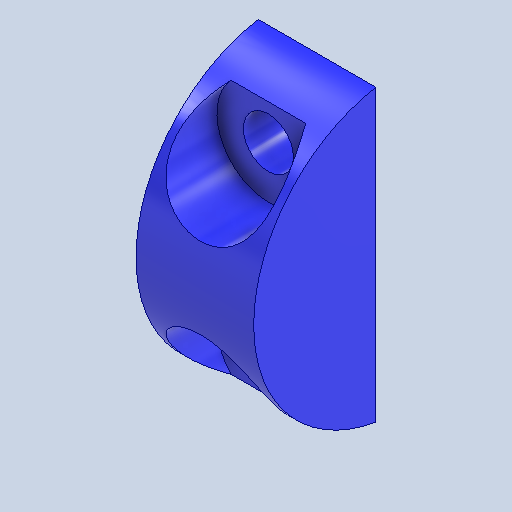
# Autodesk Inventor part: RZvector-v1-3DP-E-F
Saved by Autodesk Inventor 2025.2 (Build 292293000, 293)
## iProperties
Created: 2023-09-09
Part Number: RZvector-v1-3DP-E-F
Material: ABS プラスチック
Document SubType Name: Modeling
Designer: haruy
Density: 1.06 g/cm^3
Appearance: 青 - 壁塗料 - 光沢
Author: haruy
Autodesk Inventor part; units mm, degrees
ref_plane "YZ Plane" through (0, 0, 0) normal (1, 0, 0) x (0, 1, 0)
ref_plane "XZ Plane" through (0, 0, 0) normal (0, 1, 0) x (-1, 0, 0)
sketch "スケッチ1" plane through (0, 0, 0) normal (1, 0, 0) x (0, 1, 0)
  circle A0 centre (3.6474, 8.0868) radius 10
  circle A1 centre (3.6474, 8.0868) radius 2.1
  line L0 (2.3974, 9.7742) -> (4.8974, 9.7742)
  line L1 (-4.3526, 14.0868) -> (-4.3526, 2.0868) construction
  line L2 (-1.3526, 16.747) -> (-1.3526, -0.5735) construction
  line L3 (2.3974, 9.7742) -> (13.504, 9.7742)
  line L4 (13.504, 9.7742) -> (-6.2092, 9.7742)
  point P0 (0, 0)
  point P1 (-6.3526, 8.0868)
  dimension "d0" = 20
  dimension "d1" = 4.2
  dimension "d2" = 2.5
  dimension "d3" = 3
  dimension "d4" = 5
  constraints: 10 end point, 2 coincident, 2 point on circle, 2 point on line, 1 centre point, 1 horizontal, 1 parallel, 1 vertical, 9 other
  measures "d1" diameter of A1
  measures "d2" distance of L0.start L0.end
  measures "d3" distance between parallel lines of L1 L2
  measures "d4" distance from line of L2 point (3.647, 8.087)
extrude "押し出し1" add sketch "スケッチ1" along normal blind 8 contours L3 A1 L4 A0 | L0 A1 picked at (-3.121, 10.5193) picked at (3.6474, 9.9117)
ref_plane "作業平面1" through (0, 3.6474, 18.0868) normal (0, 0, 1) x (1, 0, 0)
sketch "スケッチ2" plane through (0, 3.6474, 18.0868) normal (0, 0, 1) x (1, 0, 0)
  circle A0 centre (4, -6.25) radius 1.7
  line L0 (8, -9.8566) -> (8, 9.8566) projected
  line L1 (0, -9.8566) -> (0, 9.8566) projected
  line L2 (0, -1.25) -> (8, -1.25)
  line L3 (8, 0) -> (0, 0)
  circle A1 centre (4, 6.25) radius 1.7
  circle A2 centre (4, -6.25) radius 3.5
  circle A3 centre (4, 6.25) radius 3.5
  point P0 (0, -3.6474)
  dimension "d7" = 3.4
  dimension "d9" = 4
  dimension "d10" = 1.25
  dimension "d11" = 5
  dimension "d14" = 7
  dimension "d15" = 7
  constraints: 4 centre point, 4 end point, 2 coincident, 2 midpoint, 2 point on line, 1 perpendicular, 1 symmetric about line, 1 other
  measures "d7" diameter of A0
  measures "d9" distance from line of A0.centre L0
  measures "d10" distance from line of L3.start L2
  measures "d11" distance from line of A0.centre L2
  measures "d14" diameter of A2
  measures "d15" diameter of A3
extrude "押し出し2" cut sketch "スケッチ2" against normal blind 15 contours A0 | A1
extrude "押し出し3" cut sketch "スケッチ2" against normal blind 5 contours A0 | A2 | A3
